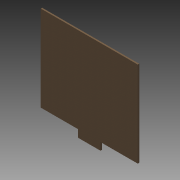
# Autodesk Inventor part: Base_Under
Saved by Autodesk Inventor 2014 SP1 (Build 180222100, 222)
## iProperties
Created: 2015-04-07
Part Number: Base_Under
Material: MDF Medium Density Fiberboard
Document SubType Name: Modeling
Designer: tuleu
Density: 0.8 g/cm^3
Appearance: Cardboard - Corrugated
Author: tuleu
Autodesk Inventor part; units mm, degrees
ref_plane "YZ Plane" through (0, 0, 0) normal (1, 0, 0) x (0, 1, 0)
ref_plane "XZ Plane" through (0, 0, 0) normal (0, 1, 0) x (-1, 0, 0)
ref_plane "XY Plane" through (0, 0, 0) normal (0, 0, 1) x (1, 0, 0)
sketch "Sketch1" plane through (0, 0, 0) normal (0, 1, 0) x (-1, 0, 0)
  line L0 (650, -625) -> (-650, -625)
  line L1 (-650, -625) -> (-650, 625)
  line L2 (-650, 625) -> (650, 625)
  line L3 (650, 625) -> (650, -625)
  line L4 (0, -625) -> (0, 625)
  line L5 (650, 0) -> (-650, 0)
  point P0 (0, 0)
  point P1 (0, 0)
  dimension "d0" = 1250
  dimension "d1" = 1300
  constraints: 12 end point, 5 midpoint, 3 perpendicular, 2 parallel, 1 coincident, 1 horizontal, 2 other
  measures "d0" distance between parallel lines of L2 L0
  measures "d1" distance of L0.start L0.end
extrude "Extrusion1" add sketch "Sketch1" along normal blind 19
sketch "Sketch2" plane through (0, 19, 0) normal (0, 1, 0) x (1, 0, 0)
  line L0 (650, 625) -> (-650, 625) projected
  line L1 (650, 625) -> (150, 625)
  line L2 (150, 625) -> (150, 525)
  line L3 (150, 525) -> (650, 525)
  line L4 (650, 525) -> (650, 625)
  line L5 (-650, 625) -> (-150, 625)
  line L6 (-150, 625) -> (-150, 525)
  line L7 (-150, 525) -> (-650, 525)
  line L8 (-650, 525) -> (-650, 625)
  line L9 (0, 525) -> (-1292.5, 525) projected
  line L10 (0, 525) -> (0, 625)
  point P0 (0, 0)
  dimension "d4" = 300
  constraints: 18 end point, 4 parallel, 2 collinear, 2 horizontal, 2 perpendicular, 1 midpoint, 1 other
  measures "d4" distance between parallel lines of L2 L6
extrude "Extrusion2" cut sketch "Sketch2" against normal up to next contours L4 L3 L2 L0 | L6 L7 L8 L0
body "Solid1"
